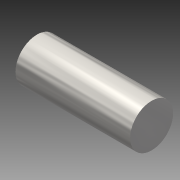
# Autodesk Inventor part: Ring1_Center_JacobMorgan_030415_pd3
Saved by Autodesk Inventor 2015 (Build 190159000, 159)
## iProperties
Created: 2015-03-04
Part Number: Ring1_Center_JacobMorgan_030415_pd3
Material: Titanium
Document SubType Name: Modeling
Designer: WASHHSST
Density: 4.51 g/cm^3
Appearance: Titanium
Author: WASHHSST
Autodesk Inventor part; units mm, degrees
ref_plane "YZ Plane" through (0, 0, 0) normal (1, 0, 0) x (0, 1, 0)
ref_plane "XZ Plane" through (0, 0, 0) normal (0, 1, 0) x (-1, 0, 0)
ref_plane "XY Plane" through (0, 0, 0) normal (0, 0, 1) x (1, 0, 0)
sketch "Sketch1" plane through (0, 0, 0) normal (1, 0, 0) x (0, 1, 0)
  circle A0 centre (0, 0) radius 9.525
  dimension "d0" = 19.05
  constraints: 1 centre point, 1 coincident
  measures "d0" diameter of A0
extrude "Extrusion1" add sketch "Sketch1" along normal blind 50.8
sketch "Sketch2" plane through (0, 0, 0) normal (-1, 0, 0) x (0, 0, 1)
  circle A0 centre (-3.4916, 3.815) radius 1.27
  circle A1 centre (3.1502, -3.8735) radius 1.27
  point P0 (0, 0)
  dimension "d4" = 2.54
  dimension "d5" = 2.54
  constraints: 2 centre point
  measures "d4" diameter of A0
  measures "d5" diameter of A1
extrude "Extrusion2" add sketch "Sketch2" along normal blind 3.81
body "Solid1"
